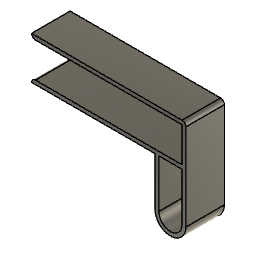
bracket v2 (Autodesk Fusion 360 design; units mm, degrees)
Autodesk Fusion 360 part; units mm, degrees
sketch "Sketch1" plane through (0, 0, 0) normal (0, 1, 0) x (1, 0, 0)
  line L0 (21, -22) -> (21, 25)
  arc A0 (21, 25) -> (5, 25) centre (13, 25) ccw
  line L1 (5, 25) -> (5, 0)
  line L2 (5, 0) -> (-59, 0)
  line L3 (-59, 0) -> (-59, -2)
  line L4 (-59, -2) -> (5, -2)
  line L5 (5, -2) -> (5, -20)
  line L6 (5, -20) -> (-59, -20)
  line L7 (-59, -20) -> (-59, -22)
  line L8 (-59, -22) -> (21, -22)
  circle A1 centre (13, 25) radius 6
  dimension "d1" = 18
  dimension "d2" = 2
  dimension "d3" = 2
  dimension "d4" = 8
  dimension "d7" = 80
  dimension "d8" = 16
  dimension "d9" = 64
  dimension "d10" = 12
  constraint vertical L0
  constraint tangent L0 A0
  constraint tangent A0 L1
  constraint parallel L0 L1
  constraint perpendicular L1 L2
  constraint perpendicular L2 L3
  constraint perpendicular L3 L4
  constraint perpendicular L4 L5
  constraint perpendicular L5 L6
  constraint perpendicular L6 L7
  constraint perpendicular L0 L8
  constraint concentric A0 A1
  measures "d1" distance of L4.end L5.end
  measures "d2" distance of L2.end L3.end
  measures "d3" distance of L6.end L7.end
  measures "d4" radius of A0
  measures "d7" distance of L0.start L7.end
  measures "d8" distance of L0 L5.end
  measures "d9" distance of L1.end L2.end
  measures "d10" diameter of A1
extrude "Extrude1" add sketch "Sketch1" along normal blind 20
sketch "Sketch2" plane through (0, 0, 0) normal (0, 1, 0) x (1, 0, 0)
  line L0 (5, -20) -> (19, -20)
  line L1 (19, -20) -> (19, -2)
  line L2 (19, -2) -> (5, -2)
  line L3 (5, -2) -> (5, -20)
  line L4 (7, 0) -> (19, 0)
  line L5 (19, 0) -> (19, 25)
  line L6 (19, 25) -> (7, 25)
  line L7 (7, 25) -> (7, 0)
  constraint horizontal L0
  constraint vertical L1
  constraint horizontal L2
  constraint vertical L3
  constraint horizontal L4
  constraint vertical L5
  constraint horizontal L6
  constraint vertical L7
extrude "Extrude2" cut sketch "Sketch2" along normal blind 23 contours L0 L1 L2 L3
sketch "Sketch3" plane through (0, 0, 0) normal (0, 1, 0) x (1, 0, 0)
  line L0 (7, 0) -> (19, 0)
  line L1 (19, 0) -> (19, 25)
  line L2 (19, 25) -> (7, 25)
  line L3 (7, 25) -> (7, 0)
  constraint horizontal L0
  constraint vertical L1
  constraint horizontal L2
  constraint vertical L3
extrude "Extrude3" cut sketch "Sketch3" along normal blind 25
fillet "Fillet1" radius 2 1 edges at (-59, 10, 20)
fillet "Fillet2" radius 2 1 edges at (-59, 10, 2)
fillet "Fillet3" radius 2 1 edges at (21, 10, 22)
